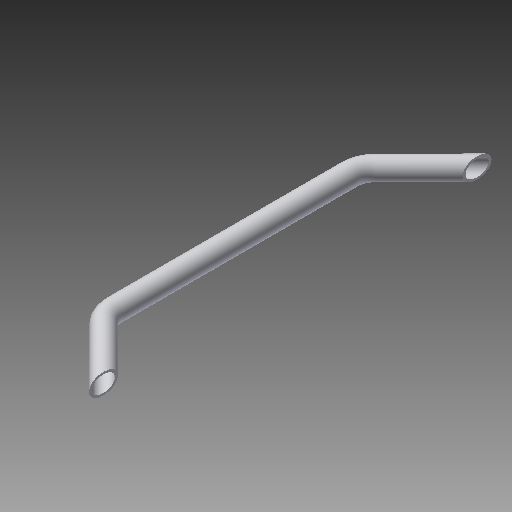
# Autodesk Inventor part: Rura_poprzeczna_wygieta
Saved by Autodesk Inventor 2017 (Build 210142000, 142)
## iProperties
Created: 2015-11-20
Part Number: Rura_poprzeczna_wygieta
Material: Aluminium AW-7020
Document SubType Name: Modelowanie
Designer: graaapsik
Density: 2.78 g/cm^3
Appearance: Aluminium AW-7020
Sheet Metal Rule: Default
Mass: 128.908 g
Surface Area: 466.898 cm^2
Volume: 46.3699 cm^3
Author: graaapsik
Autodesk Inventor part; units mm, degrees
note: some values were not read from the file. Chosen so that the rebuilt part matches the saved one: bend side of "Gięcie części2".
ref_plane "YZ Plane" through (0, 0, 0) normal (1, 0, 0) x (0, 1, 0)
ref_plane "XZ Plane" through (0, 0, 0) normal (0, 1, 0) x (-1, 0, 0)
ref_plane "XY Plane" through (0, 0, 0) normal (0, 0, 1) x (1, 0, 0)
sketch "Szkic1" plane through (0, 0, 0) normal (0, 0, 1) x (1, 0, 0)
  circle A0 centre (0, 0) radius 10
  dimension "d0" = 20
  constraints: 1 centre point, 1 coincident
  measures "d0" diameter of A0
extrude "Wyciągnięcie proste1" add sketch "Szkic1" along normal blind 430
shell "Skorupa1" thickness 2 removed faces 2 at (-1.182, 3.1167, 430) at (-1.182, 3.1167, 0)
sketch "Szkic2" plane through (0, 0, 0) normal (1, 0, 0) x (0, 1, 0)
  line L0 (-34.5081, 100) -> (42.8278, 100)
  line L1 (-10, 0) -> (10, 0) projected
  line L2 (10, 430) -> (-10, 430) projected
  point P0 (0, 0)
  dimension "d4" = 100
  constraints: 2 end point, 1 horizontal
  measures "d4" distance from line of L0.start L1
bend part "Gięcie części1" radius 25.4648 angle 45 line through (0, -34.5081, 100) along (0, 1, 0) centre toward (1, 0, 0) moving side (0, 0, -1) both sides no
sketch "Szkic3" plane through (0, 0, 0) normal (1, 0, 0) x (0, 1, 0)
  line L0 (-35.2697, 330) -> (39.6293, 330)
  line L1 (10, 430) -> (-10, 430) projected
  point P0 (0, 0)
  dimension "d8" = 100
  constraints: 2 end point, 1 horizontal
  measures "d8" distance between parallel lines of L0 L1
bend part "Gięcie części2" radius 25.4648 angle 45 line through (0, -35.2697, 330) along (0, 1, 0) centre toward (1, 0, 0) moving side (0, 0, 1) both sides no
sketch "Szkic4" plane through (0, 0, 0) normal (0, 1, 0) x (-1, 0, 0)
  line L0 (-71.0981, 32.4962) -> (-56.9559, 18.3541) construction
  line L1 (-56.9559, 18.3541) -> (-0.3874, 74.9226) construction
  line L2 (-56.9559, 18.3541) -> (-56.9559, 46.6383)
  line L3 (-71.0981, 32.4962) -> (-14.5295, 89.0647) construction
  line L4 (-56.9559, 46.6383) -> (-71.0981, 32.4962)
  line L5 (-71.0981, 32.4962) -> (-56.9559, 18.3541)
  line L6 (-56.9559, 411.6459) -> (-71.0981, 397.5038) construction
  line L7 (-14.5295, 340.9353) -> (-71.0981, 397.5038) construction
  line L8 (-0.3874, 355.0774) -> (-56.9559, 411.6459) construction
  line L9 (-56.9559, 411.6459) -> (-56.9559, 383.3617)
  line L10 (-56.9559, 383.3617) -> (-71.0981, 397.5038)
  line L11 (-71.0981, 397.5038) -> (-56.9559, 411.6459)
  point P0 (0, 0)
  constraints: 12 end point, 5 collinear, 2 point on line, 1 vertical
extrude "Wyciągnięcie proste3" cut sketch "Szkic4" along normal mid plane 32
equation "\"PromieńGięcia\" = Grubość"
equation "\"SzerokośćGięciaPodcięcia\" = Grubość"
equation "\"GłębokośćGięciaPodcięcia\" = 0.5 * Grubość"
equation "\"RozmiarPodcięciaNarożnika\" = 4 * Grubość"
equation "\"MinimalnaPozostałość\" = 2 * Grubość"
equation "\"PromieńPrzejścia\" = PromieńGięcia"
equation "\"Rozmiar_promienia_Jacobiego\" = Grubość"
equation "\"Wielk_odstępu\" = Grubość"
equation "\"Grubość\" = 0.5"
